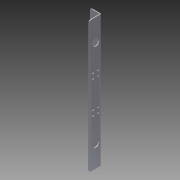
# Autodesk Inventor part: V5 Shooter Frame Channel Part 1
Saved by Autodesk Inventor 2014 SP1 (Build 180222100, 222)
## iProperties
Created: 2012-01-30
Part Number: V5 Shooter Frame Channel Part 1
Material: Aluminum-6061
Document SubType Name: Sheet Metal
Designer: Moses
Density: 2.71 g/cm^3
Sheet Metal Rule: Default
Mass: 348.647 g
Surface Area: 866.817 cm^2
Volume: 128.652 cm^3
Flat Pattern Width: 50.8 cm
Flat Pattern Length: 8.34697 cm
Flat Pattern Area: 424.026 cm^2
Sheet Metal Width: 20.000 in
Sheet Metal Length: 3.286 in
Sheet Metal Area: 65.724 in^2
Appearance: Aluminum - Flat
p1holedistedge: 0.550 in
d34: 0.750 in
p1mountholedia: 0.266 in
p1holespacing: 0.750 in
Author: Moses
Autodesk Inventor part; units mm, degrees
ref_plane "YZ Plane" through (0, 0, 0) normal (1, 0, 0) x (0, 1, 0)
ref_plane "XZ Plane" through (0, 0, 0) normal (0, 1, 0) x (-1, 0, 0)
sketch "Sketch1" plane through (0, 0, 0) normal (0, 0, 1) x (1, 0, 0)
  line L0 (0, 0) -> (81.0608, 0)
  line L1 (0, 0) -> (0, 508)
  line L2 (0, 508) -> (81.0608, 508)
  line L3 (81.0608, 508) -> (81.0608, 0)
  line L4 (36.6108, 508) -> (36.6108, 0) construction
  line L5 (36.4838, 6.35) -> (36.7378, 6.35)
  line L6 (36.4838, 6.35) -> (36.4838, 12.7)
  line L7 (36.4838, 12.7) -> (36.7378, 12.7)
  line L8 (36.7378, 12.7) -> (36.7378, 6.35)
  line L9 (36.4838, 23.2103) -> (36.7378, 23.2103)
  line L10 (36.4838, 23.2103) -> (36.4838, 29.5603)
  line L11 (36.4838, 29.5603) -> (36.7378, 29.5603)
  line L12 (36.7378, 29.5603) -> (36.7378, 23.2103)
  line L13 (36.4838, 40.0707) -> (36.7378, 40.0707)
  line L14 (36.4838, 40.0707) -> (36.4838, 46.4207)
  line L15 (36.4838, 46.4207) -> (36.7378, 46.4207)
  line L16 (36.7378, 46.4207) -> (36.7378, 40.0707)
  line L17 (36.4838, 56.931) -> (36.7378, 56.931)
  line L18 (36.4838, 56.931) -> (36.4838, 63.281)
  line L19 (36.4838, 63.281) -> (36.7378, 63.281)
  line L20 (36.7378, 63.281) -> (36.7378, 56.931)
  line L21 (36.4838, 73.7914) -> (36.7378, 73.7914)
  line L22 (36.4838, 73.7914) -> (36.4838, 80.1414)
  line L23 (36.4838, 80.1414) -> (36.7378, 80.1414)
  line L24 (36.7378, 80.1414) -> (36.7378, 73.7914)
  line L25 (36.4838, 90.6517) -> (36.7378, 90.6517)
  line L26 (36.4838, 90.6517) -> (36.4838, 97.0017)
  line L27 (36.4838, 97.0017) -> (36.7378, 97.0017)
  line L28 (36.7378, 97.0017) -> (36.7378, 90.6517)
  line L29 (36.4838, 107.5121) -> (36.7378, 107.5121)
  line L30 (36.4838, 107.5121) -> (36.4838, 113.8621)
  line L31 (36.4838, 113.8621) -> (36.7378, 113.8621)
  line L32 (36.7378, 113.8621) -> (36.7378, 107.5121)
  line L33 (36.4838, 124.3724) -> (36.7378, 124.3724)
  line L34 (36.4838, 124.3724) -> (36.4838, 130.7224)
  line L35 (36.4838, 130.7224) -> (36.7378, 130.7224)
  line L36 (36.7378, 130.7224) -> (36.7378, 124.3724)
  line L37 (36.4838, 141.2328) -> (36.7378, 141.2328)
  line L38 (36.4838, 141.2328) -> (36.4838, 147.5828)
  line L39 (36.4838, 147.5828) -> (36.7378, 147.5828)
  line L40 (36.7378, 147.5828) -> (36.7378, 141.2328)
  line L41 (36.4838, 158.0931) -> (36.7378, 158.0931)
  line L42 (36.4838, 158.0931) -> (36.4838, 164.4431)
  line L43 (36.4838, 164.4431) -> (36.7378, 164.4431)
  line L44 (36.7378, 164.4431) -> (36.7378, 158.0931)
  line L45 (36.4838, 174.9534) -> (36.7378, 174.9534)
  line L46 (36.4838, 174.9534) -> (36.4838, 181.3034)
  line L47 (36.4838, 181.3034) -> (36.7378, 181.3034)
  line L48 (36.7378, 181.3034) -> (36.7378, 174.9534)
  line L49 (36.4838, 191.8138) -> (36.7378, 191.8138)
  line L50 (36.4838, 191.8138) -> (36.4838, 198.1638)
  line L51 (36.4838, 198.1638) -> (36.7378, 198.1638)
  line L52 (36.7378, 198.1638) -> (36.7378, 191.8138)
  line L53 (36.4838, 208.6741) -> (36.7378, 208.6741)
  line L54 (36.4838, 208.6741) -> (36.4838, 215.0241)
  line L55 (36.4838, 215.0241) -> (36.7378, 215.0241)
  line L56 (36.7378, 215.0241) -> (36.7378, 208.6741)
  line L57 (36.4838, 225.5345) -> (36.7378, 225.5345)
  line L58 (36.4838, 225.5345) -> (36.4838, 231.8845)
  line L59 (36.4838, 231.8845) -> (36.7378, 231.8845)
  line L60 (36.7378, 231.8845) -> (36.7378, 225.5345)
  line L61 (36.4838, 242.3948) -> (36.7378, 242.3948)
  line L62 (36.4838, 242.3948) -> (36.4838, 248.7448)
  line L63 (36.4838, 248.7448) -> (36.7378, 248.7448)
  line L64 (36.7378, 248.7448) -> (36.7378, 242.3948)
  line L65 (36.4838, 259.2552) -> (36.7378, 259.2552)
  line L66 (36.4838, 259.2552) -> (36.4838, 265.6052)
  line L67 (36.4838, 265.6052) -> (36.7378, 265.6052)
  line L68 (36.7378, 265.6052) -> (36.7378, 259.2552)
  line L69 (36.4838, 276.1155) -> (36.7378, 276.1155)
  line L70 (36.4838, 276.1155) -> (36.4838, 282.4655)
  line L71 (36.4838, 282.4655) -> (36.7378, 282.4655)
  line L72 (36.7378, 282.4655) -> (36.7378, 276.1155)
  line L73 (36.4838, 292.9759) -> (36.7378, 292.9759)
  line L74 (36.4838, 292.9759) -> (36.4838, 299.3259)
  line L75 (36.4838, 299.3259) -> (36.7378, 299.3259)
  line L76 (36.7378, 299.3259) -> (36.7378, 292.9759)
  line L77 (36.4838, 309.8362) -> (36.7378, 309.8362)
  line L78 (36.4838, 309.8362) -> (36.4838, 316.1862)
  line L79 (36.4838, 316.1862) -> (36.7378, 316.1862)
  line L80 (36.7378, 316.1862) -> (36.7378, 309.8362)
  line L81 (36.4838, 326.6966) -> (36.7378, 326.6966)
  line L82 (36.4838, 326.6966) -> (36.4838, 333.0466)
  line L83 (36.4838, 333.0466) -> (36.7378, 333.0466)
  line L84 (36.7378, 333.0466) -> (36.7378, 326.6966)
  line L85 (36.4838, 343.5569) -> (36.7378, 343.5569)
  line L86 (36.4838, 343.5569) -> (36.4838, 349.9069)
  line L87 (36.4838, 349.9069) -> (36.7378, 349.9069)
  line L88 (36.7378, 349.9069) -> (36.7378, 343.5569)
  line L89 (36.4838, 360.4172) -> (36.7378, 360.4172)
  line L90 (36.4838, 360.4172) -> (36.4838, 366.7672)
  line L91 (36.4838, 366.7672) -> (36.7378, 366.7672)
  line L92 (36.7378, 366.7672) -> (36.7378, 360.4172)
  line L93 (36.4838, 377.2776) -> (36.7378, 377.2776)
  line L94 (36.4838, 377.2776) -> (36.4838, 383.6276)
  line L95 (36.4838, 383.6276) -> (36.7378, 383.6276)
  line L96 (36.7378, 383.6276) -> (36.7378, 377.2776)
  line L97 (36.4838, 394.1379) -> (36.7378, 394.1379)
  line L98 (36.4838, 394.1379) -> (36.4838, 400.4879)
  line L99 (36.4838, 400.4879) -> (36.7378, 400.4879)
  line L100 (36.7378, 400.4879) -> (36.7378, 394.1379)
  line L101 (36.4838, 410.9983) -> (36.7378, 410.9983)
  line L102 (36.4838, 410.9983) -> (36.4838, 417.3483)
  line L103 (36.4838, 417.3483) -> (36.7378, 417.3483)
  line L104 (36.7378, 417.3483) -> (36.7378, 410.9983)
  line L105 (36.4838, 427.8586) -> (36.7378, 427.8586)
  line L106 (36.4838, 427.8586) -> (36.4838, 434.2086)
  line L107 (36.4838, 434.2086) -> (36.7378, 434.2086)
  line L108 (36.7378, 434.2086) -> (36.7378, 427.8586)
  line L109 (36.4838, 444.719) -> (36.7378, 444.719)
  line L110 (36.4838, 444.719) -> (36.4838, 451.069)
  line L111 (36.4838, 451.069) -> (36.7378, 451.069)
  line L112 (36.7378, 451.069) -> (36.7378, 444.719)
  line L113 (36.4838, 461.5793) -> (36.7378, 461.5793)
  line L114 (36.4838, 461.5793) -> (36.4838, 467.9293)
  line L115 (36.4838, 467.9293) -> (36.7378, 467.9293)
  line L116 (36.7378, 467.9293) -> (36.7378, 461.5793)
  line L117 (36.4838, 478.4397) -> (36.7378, 478.4397)
  line L118 (36.4838, 478.4397) -> (36.4838, 484.7897)
  line L119 (36.4838, 484.7897) -> (36.7378, 484.7897)
  line L120 (36.7378, 484.7897) -> (36.7378, 478.4397)
  line L121 (36.4838, 495.3) -> (36.7378, 495.3)
  line L122 (36.4838, 495.3) -> (36.4838, 501.65)
  line L123 (36.4838, 501.65) -> (36.7378, 501.65)
  line L124 (36.7378, 501.65) -> (36.7378, 495.3)
  line L125 (-2.4088, 400.045) -> (-2.4088, 447.045) projected
  line L126 (-2.4088, 60.955) -> (-2.4088, 107.955) projected
  line L127 (-2.4088, 107.955) -> (-2.4088, 400.045)
  line L128 (-2.4088, 447.045) -> (-2.4088, 508)
  line L129 (-2.4088, 508) -> (0, 508)
  line L130 (-2.4088, 60.955) -> (-2.4088, 0)
  line L131 (-2.4088, 0) -> (0, 0)
  line L132 (14.3858, 508) -> (14.3858, 0) construction
  circle A0 centre (14.3858, 127) radius 11.1125
  circle A1 centre (14.3858, 163.2857) radius 11.1125
  circle A2 centre (14.3858, 199.5714) radius 11.1125
  circle A3 centre (14.3858, 235.8571) radius 11.1125
  circle A4 centre (14.3858, 272.1429) radius 11.1125
  circle A5 centre (14.3858, 308.4286) radius 11.1125
  circle A6 centre (14.3858, 344.7143) radius 11.1125
  circle A7 centre (14.3858, 381) radius 11.1125
  point P0 (36.6108, 12.7)
  point P1 (36.6108, 29.5603)
  point P2 (36.6108, 46.4207)
  point P3 (36.6108, 63.281)
  point P4 (36.6108, 80.1414)
  point P5 (36.6108, 97.0017)
  point P6 (36.6108, 113.8621)
  point P7 (36.6108, 130.7224)
  point P8 (36.6108, 147.5828)
  point P9 (36.6108, 164.4431)
  point P10 (36.6108, 181.3034)
  point P11 (36.6108, 198.1638)
  point P12 (36.6108, 215.0241)
  point P13 (36.6108, 231.8845)
  point P14 (36.6108, 248.7448)
  point P15 (36.6108, 265.6052)
  point P16 (36.6108, 282.4655)
  point P17 (36.6108, 299.3259)
  point P18 (36.6108, 316.1862)
  point P19 (36.6108, 333.0466)
  point P20 (36.6108, 349.9069)
  point P21 (36.6108, 366.7672)
  point P22 (36.6108, 383.6276)
  point P23 (36.6108, 400.4879)
  point P24 (36.6108, 417.3483)
  point P25 (36.6108, 434.2086)
  point P26 (36.6108, 451.069)
  point P27 (36.6108, 467.9293)
  point P28 (36.6108, 484.7897)
  point P29 (36.6108, 501.65)
  dimension "d0" = 81.0608
  dimension "d1" = 508
  dimension "d2" = 44.45
  dimension "d3" = 0.254
  dimension "d4" = 6.35
  dimension "d5" = 6.35
  dimension "d8" = 16.8603
  dimension "d82" = 22.225
  dimension "d83" = 22.225
  dimension "d84" = 127
  dimension "d87" = 36.2857
  constraints: 262 end point, 11 perpendicular, 8 centre point, 6 point on line, 2 parallel, 2 vertical, 1 collinear, 1 horizontal, 1 midpoint, 275 other
  measures "d0" distance of L0.start L0.end
  measures "d1" distance of L0.start L1.end
  measures "d2" distance between parallel lines of L3 L4
  measures "d3" distance of L5.start L5.end
  measures "d4" distance of L5.start L6.end
  measures "d5" distance between parallel lines of L0 L5
  measures "d8" distance of L5.start L10.start
  measures "d82" distance between parallel lines of L4 L132
  measures "d83" diameter of A0
  measures "d84" distance from line of L0 A0.centre
  measures "d87" distance of A0.centre A1.centre
extrude "Plate1" add sketch "Sketch1" along normal blind 3.175 contours L1 L2 L3 L0 | L131 L130 L126 L127 L125 L128 L129 L1 | L6 L7 L8 L5 | L10 L11 L12 L9 | L14 L15 L16 L13 | L18 L19 L20 L17 | L22 L23 L24 L21 | L26 L27 L28 L25 | L30 L31 L32 L29 | L34 L35 L36 L33 | L38 L39 L40 L37 | L42 L43 L44 L41 | L46 L47 L48 L45 | L50 L51 L52 L49 | L54 L55 L56 L53 | L58 L59 L60 L57 | L62 L63 L64 L61 | L66 L67 L68 L65 | L70 L71 L72 L69 | L74 L75 L76 L73 | L78 L79 L80 L77 | L82 L83 L84 L81 | L86 L87 L88 L85 | L90 L91 L92 L89 | L94 L95 L96 L93 | L98 L99 L100 L97 | L102 L103 L104 L101 | L106 L107 L108 L105 | L110 L111 L112 L109 | L114 L115 L116 L113 | L118 L119 L120 L117 | L122 L123 L124 L121 | A0 | A1 | A2 | A3 | A4 | A5 | A6 | A7
fold "Fold1" angle 90 bend radius 1.27 thickness 3.175 k factor 0.44 line from (36.6108, 508, 0) to (36.6108, 0, 0) line at bend centre moving side (1, 0, 0) folds toward (0, 0, 1)
sketch "Sketch2" plane through (38.9612, 0, 46.8003) normal (1, 0, 0) x (0, 0, -1)
  line L0 (0, 0) -> (0, 508) projected
  line L1 (46.8003, 508) -> (46.8003, 0) projected
  circle A0 centre (24.5753, 423.545) radius 14.2875
  line L2 (0, 254) -> (46.8003, 254) construction
  circle A1 centre (24.5753, 84.455) radius 14.2875
  dimension "d20" = 28.575
  dimension "d21" = 22.225
  dimension "d22" = 339.09
  constraints: 2 centre point, 2 end point, 2 midpoint, 1 symmetric about line, 1 other
  measures "d20" diameter of A0
  measures "d21" distance from line of L1 A0.centre
  measures "d22" distance of A0.centre A1.centre
extrude "Cut1" cut sketch "Sketch2" against normal blind 3.175
sketch "Sketch3" plane through (0, 0, 0) normal (0, 0, -1) x (-1, 0, 0)
  line L0 (-38.9612, 0) -> (-38.9612, 508) projected
  circle A0 centre (-24.9912, 494.03) radius 3.3782
  circle A1 centre (-5.9412, 474.98) radius 3.3782
  line L1 (2.4088, 254) -> (-38.9612, 254) construction
  circle A2 centre (-30.0712, 433.07) radius 3.3782
  circle A3 centre (-24.9912, 13.97) radius 3.3782
  circle A4 centre (-5.9412, 33.02) radius 3.3782
  line L2 (-3.4012, 433.07) -> (-3.4012, 414.02) construction
  line L3 (-3.4012, 93.98) -> (-3.4012, 74.93) construction
  line L4 (-30.0712, 433.07) -> (-30.0712, 414.02) construction
  line L5 (-30.0712, 414.02) -> (-30.0712, 423.545) construction
  line L6 (-3.4012, 423.545) -> (-30.0712, 423.545) construction
  line L7 (-30.0712, 74.93) -> (-30.0712, 93.98) construction
  line L8 (-30.0712, 84.455) -> (-3.4012, 84.455) construction
  line L9 (2.4088, 508) -> (2.4088, 0) projected
  line L10 (-34.5162, 508) -> (2.4088, 508) projected
  circle A5 centre (-3.4012, 433.07) radius 3.3782
  circle A6 centre (-30.0712, 414.02) radius 3.3782
  circle A7 centre (-3.4012, 414.02) radius 3.3782
  line L11 (-30.0712, 433.07) -> (-30.0712, 414.02) construction
  line L12 (-30.0712, 414.02) -> (-30.0712, 433.07) construction
  circle A8 centre (-30.0712, 74.93) radius 3.3782
  circle A9 centre (-3.4012, 74.93) radius 3.3782
  circle A10 centre (-30.0712, 93.98) radius 3.3782
  circle A11 centre (-3.4012, 93.98) radius 3.3782
  dimension "p1mountholedia" = 6.7564
  dimension "d26" = 6.7564
  dimension "d34" = 19.05
  dimension "d35" = 6.7564
  dimension "d38" = 26.67
  dimension "d44" = 339.09
  dimension "p1holespacing" = 19.05
  dimension "d51" = 13.97
  dimension "d72" = 13.97
  dimension "d75" = 26.67
  dimension "d78" = 19.05
  dimension "d81" = 8.89
  constraints: 20 end point, 12 centre point, 9 symmetric about line, 6 midpoint, 4 perpendicular, 3 equal length, 1 coincident, 1 horizontal, 1 point on line, 1 vertical, 12 other
  measures "p1mountholedia" diameter of A0
  measures "d26" diameter of A1
  measures "d34" horizontal distance of A1.centre A0.centre
  measures "d35" diameter of A2
  measures "d38" distance of L4.start L2.start
  measures "d44" distance between parallel lines of L6 L8
  measures "p1holespacing" horizontal distance of A1.centre A0.centre
  measures "d51" distance from line of L0 A0.centre
  measures "d72" distance from line of L10 A0.centre
  measures "d75" distance of L4.start A5.centre
  measures "d78" distance of L4.start L11.end
  measures "d81" distance between parallel lines of L0 L4
extrude "Cut2" cut sketch "Sketch3" against normal blind 3.175
ref_plane "Work Plane1" through (38.9612, 254, 46.8003) normal (0, 1, 0) x (1, 0, 0)
fillet "Corner Round1" radius 6.35 2 edges at (37.3737, 508, 46.8003) (37.3737, 0, 46.8003)
sketch "Sketch4" plane through (38.9612, 0, 4.445) normal (1, 0, 0) x (0, 0, -1)
  line L0 (0, 0) -> (0, 508) projected
  line L1 (-42.3553, 6.35) -> (-42.3553, 501.65) projected
  line L2 (-42.3553, 254) -> (0, 254) construction
  circle A0 centre (-27.305, 306.5463) radius 3.3782
  line L3 (-27.305, 306.5463) -> (-8.255, 306.5463) construction
  circle A1 centre (-8.255, 306.5463) radius 3.3782
  circle A2 centre (-27.305, 201.4538) radius 3.3782
  circle A3 centre (-8.255, 201.4538) radius 3.3782
  line L4 (-17.78, 185.5788) -> (-17.78, 198.2788) projected
  line L5 (-17.78, 309.7213) -> (-17.78, 322.4213) projected
  line L6 (-42.3553, 316.0713) -> (0, 316.0713) construction
  circle A4 centre (-27.305, 325.5963) radius 3.3782
  circle A5 centre (-8.255, 325.5963) radius 3.3782
  line L7 (-42.3553, 191.9288) -> (0, 191.9288) construction
  line L8 (-27.305, 201.4538) -> (-8.255, 201.4538) construction
  circle A6 centre (-27.305, 182.4038) radius 3.3782
  circle A7 centre (-8.255, 182.4038) radius 3.3782
  point P0 (-42.3553, 3.175)
  point P1 (-42.3553, 504.825)
  point P2 (4.445, 0)
  point P3 (-17.78, 316.0713)
  point P4 (-17.78, 306.5463)
  point P5 (-17.78, 191.9288)
  point P6 (-17.78, 201.4538)
  dimension "d54" = 6.7564
  dimension "d55" = 6.7564
  dimension "d57" = 19.05
  dimension "d58" = 6.7564
  dimension "d60" = 6.7564
  dimension "d64" = 9.525
  dimension "d69" = 19.05
  dimension "d70" = 9.525
  constraints: 10 end point, 8 centre point, 8 point on line, 6 midpoint, 4 symmetric about line, 2 perpendicular, 1 coincident, 1 horizontal, 1 parallel, 4 other
  measures "d54" diameter of A0
  measures "d55" diameter of A1
  measures "d57" distance of L3.start L3.end
  measures "d58" diameter of A2
  measures "d60" diameter of A3
  measures "d64" distance between parallel lines of L6 L3
  measures "d69" distance of L8.start L8.end
  measures "d70" distance between parallel lines of L7 L8
extrude "Cut3" cut sketch "Sketch4" against normal blind 3.175
fillet "Corner Round2" radius 6.35 2 edges at (-2.4088, 0, 1.5875) (-2.4088, 508, 1.5875)
equation "\"d14\" = BendReliefWidth"
equation "\"d15\" = BendReliefDepth"
equation "\"d16\" = MinimumRemnant"
equation "\"d17\" = BendRadius"
equation "\"d23\" = Thickness"
equation "\"d26\" = p1mountholedia"
equation "\"d34\" = p1holespacing"
equation "\"d35\" = p1mountholedia"
equation "\"d51\" = p1holedistedge"
equation "\"d46\" = Thickness"
equation "\"BendRadius\" = Thickness"
equation "\"BendReliefWidth\" = Thickness"
equation "\"BendReliefDepth\" = 0.5 * Thickness"
equation "\"CornerReliefSize\" = 4 * Thickness"
equation "\"MinimumRemnant\" = 2 * Thickness"
equation "\"TransitionRadius\" = BendRadius"
equation "\"JacobiRadiusSize\" = BendRadius"
equation "\"GapSize\" = Thickness"
equation "\"d13\" = BendRadius"
equation "\"Thickness\" = 3.175"
equation "\"p1holedistedge\" = 13.97"
body "Solid1"
